Autodesk Inventor part; units mm, degrees
(part 2 of 2)
extrude "Extrusion4" cut sketch "Sketch4" against normal blind 2 contours A11 L20 A10 L19 L18 A9 L17 A8 L16 L25 L11 L10 L9 A5 L8 A4 L7 L6 A3 L5 A2 L4 L3 A1 L2 A0 L1 L24 L23 A13 L22 A12 L21 L0
fillet "Fillet1" radius 4 4 edges at (-72.1915, 62.8097, 3.5) (-88.7804, -31.274, 3.5) (198.4911, 62.8097, 3.5) (215.0786, -31.2745, 3.5)
fillet "Fillet2" radius 4 10 edges at (-71.4063, 61.8738, 7) (-80.4411, 16.0224, 7) (-87.4817, -30.3953, 7) (-30.1108, -43.5751, 7) (197.7059, 61.8738, 7) (206.74, 16.0221, 7) (213.7798, -30.3958, 7) (156.4089, -43.5753, 7) (63.1498, 62.8097, 7) (63.149, -55.0813, 7)
fillet "Fillet3" radius 1 28 edges at (-62.9014, 53.3064, 4.5) (-24.9574, 49.6622, 4.5) (-5.3778, 51.287, 4.5) (14.5153, 47.7794, 4.5) (32.1848, 38.5712, 4.5) (50.0279, 30.3479, 4.5) (-76.3066, -22.7207, 4.5) (-37.702, -29.5275, 4.5) (-18.5275, -29.8623, 4.5) (36.6224, -45.6793, 4.5) (16.7292, -42.1717, 4.5) (-1.1139, -33.9484, 4.5) (70.4439, -46.0074, 4.5) (89.6759, -45.6797, 4.5) (109.5691, -42.1725, 4.5) (127.4123, -33.9494, 4.5) (144.826, -29.8637, 4.5) (164.0005, -29.5291, 4.5) (202.6052, -22.723, 4.5) (189.2012, 53.3044, 4.5) (151.2572, 49.6608, 4.5) (131.6776, 51.2859, 4.5) (111.7844, 47.7786, 4.5) (94.1148, 38.5707, 4.5) (76.2716, 30.3477, 4.5) (63.6397, -7.4141, 4.5) (62.6592, -7.4141, 4.5) (55.8544, -46.0073, 4.5)
sketch "Sketch6" plane through (0, 0, 0) normal (0, 0, -1) x (-1, 0, 0)
  circle A0 centre (68.8351, 58.8097) radius 2 projected
  circle A1 centre (84.1686, -28.1539) radius 2 projected
  circle A2 centre (-31.0902, -52.3194) radius 2 projected
  circle A3 centre (84.1686, -28.1539) radius 2 projected
  circle A4 centre (-31.092, 58.8102) radius 2 projected
  circle A5 centre (-95.208, -52.3199) radius 2 projected
  circle A6 centre (-195.1347, 58.8097) radius 2 projected
  circle A7 centre (-210.4668, -28.1544) radius 2 projected
  circle A8 centre (-95.208, 58.8097) radius 2 projected
  circle A9 centre (-31.0902, -52.3194) radius 2 projected
  circle A10 centre (68.8351, 58.8097) radius 2 projected
  arc A11 (84.9894, -32.0688) -> (88.1078, -27.4594) centre (84.1686, -28.1539) ccw projected
  line L0 (72.7744, 59.5042) -> (88.1078, -27.4594) projected
  arc A12 (72.7744, 59.5042) -> (68.8351, 62.8097) centre (68.8351, 58.8097) ccw projected
  line L1 (-195.1347, 62.8097) -> (68.8351, 62.8097) projected
  arc A13 (-195.1347, 62.8097) -> (-199.0739, 59.5042) centre (-195.1347, 58.8097) ccw projected
  line L2 (-214.4061, -27.4599) -> (-199.0739, 59.5042) projected
  arc A14 (-214.4061, -27.4599) -> (-211.2876, -32.0693) centre (-210.4668, -28.1544) ccw projected
  line L3 (-101.5302, -55.0813) -> (-211.2876, -32.0693) projected
  line L4 (-24.7678, -55.0813) -> (-101.5302, -55.0813) projected
  line L5 (84.9894, -32.0688) -> (-24.7678, -55.0813) projected
  point P0 (0, 0)
hole "Hole2" at (195.1347, 58.8097, 0) at (210.4668, -28.1544, 0) at (95.208, -52.3199, 0) at (31.0902, -52.3194, 0) at (95.208, 58.8097, 0) at (31.092, 58.8102, 0) at (-84.1686, -28.1539, 0) at (-68.8351, 58.8097, 0) direction (0, 0, 1) diameter 2 depth 4 tip angle 118
equation "\"d9\" = d8"
equation "\"d10\" = d8"
equation "\"d11\" = d8"
equation "\"d12\" = d8"
equation "\"d13\" = d8"
equation "\"d14\" = d8"
equation "\"d15\" = d8"
equation "\"d16\" = d8"
equation "\"d17\" = d8"
equation "\"d18\" = d8"
equation "\"d19\" = d8"
equation "\"d20\" = d8"
equation "\"d21\" = d8"
equation "\"d22\" = d8"
equation "\"d23\" = d8"
equation "\"d24\" = d8"
equation "\"d25\" = d8"
equation "\"d26\" = d8"
equation "\"d27\" = d8"
equation "\"d28\" = d8"
equation "\"d32\" = d8"
equation "\"d33\" = d8"
equation "\"d34\" = d8"
equation "\"d1\" = d0"
equation "\"d3\" = d0"
equation "\"d4\" = d0"
equation "\"d5\" = d0"
equation "\"d0\" = 9"
body "Solid1"
